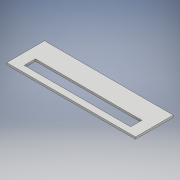
# Autodesk Inventor part: frontpannel
Saved by Autodesk Inventor 2017 (Build 210142000, 142)
## iProperties
Created: 2016-10-21
Part Number: frontpannel
Material: Generic
Document SubType Name: Sheet Metal
Designer: aesen
Density: 1 g/cm^3
Sheet Metal Rule: Default_mm
Appearance: Default
Author: aesen
Autodesk Inventor part; units mm, degrees
ref_plane "YZ Plane" through (0, 0, 0) normal (1, 0, 0) x (0, 1, 0)
ref_plane "XZ Plane" through (0, 0, 0) normal (0, 1, 0) x (-1, 0, 0)
ref_plane "XY Plane" through (0, 0, 0) normal (0, 0, 1) x (1, 0, 0)
sketch "Sketch1" plane through (0, 0, 0) normal (0, 0, 1) x (1, 0, 0)
  line L0 (-12.0469, 112.9187) -> (390.8479, 112.9187)
  line L1 (390.8479, 112.9187) -> (390.8479, -5.3691)
  line L2 (390.8479, -5.3691) -> (-12.0469, -5.3691)
  line L3 (-12.0469, -5.3691) -> (-12.0469, 112.9187)
  line L4 (22.9531, 49.6309) -> (355.8479, 49.6309)
  line L5 (355.8479, 49.6309) -> (355.8479, 14.6309)
  line L6 (355.8479, 14.6309) -> (22.9531, 14.6309)
  line L7 (22.9531, 14.6309) -> (22.9531, 49.6309)
  point P0 (0, 0)
  dimension "d0" = 402.8948
  dimension "d1" = 118.2878
  dimension "d4" = 35
  dimension "d5" = 35
  dimension "d6" = 20
  dimension "d7" = 35
  constraints: 16 end point, 4 parallel, 2 horizontal, 2 perpendicular
  measures "d0" distance between parallel lines of L1 L3
  measures "d1" distance between parallel lines of L2 L0
  measures "d4" distance between parallel lines of L7 L3
  measures "d5" distance between parallel lines of L1 L5
  measures "d6" distance between parallel lines of L2 L6
  measures "d7" distance between parallel lines of L6 L4
extrude "Extrusion2" add sketch "Sketch1" along normal blind 6.35
equation "\"BendRadius\" = Thickness"
equation "\"BendReliefWidth\" = Thickness"
equation "\"BendReliefDepth\" = 0.5 * Thickness"
equation "\"CornerReliefSize\" = 4 * Thickness"
equation "\"MinimumRemnant\" = 2 * Thickness"
equation "\"TransitionRadius\" = BendRadius"
equation "\"JacobiRadiusSize\" = BendRadius"
equation "\"GapSize\" = Thickness"
equation "\"Thickness\" = 0.5"
body "Solid2"
